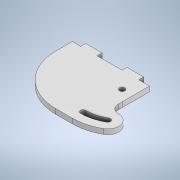
# Autodesk Inventor part: camMount
Saved by Autodesk Inventor 2020 (Build 240168000, 168)
## iProperties
Created: 2019-08-06
Part Number: camMount
Material: Generic
Document SubType Name: Modeling
Designer: n10208577
Density: 1 g/cm^3
Appearance: Default
Author: n10208577
Autodesk Inventor part; units mm, degrees
ref_plane "YZ Plane" through (0, 0, 0) normal (1, 0, 0) x (0, 1, 0)
ref_plane "XZ Plane" through (0, 0, 0) normal (0, 1, 0) x (-1, 0, 0)
ref_plane "XY Plane" through (0, 0, 0) normal (0, 0, 1) x (1, 0, 0)
sketch "Sketch1" plane through (0, 0, 0) normal (0, 1, 0) x (-1, 0, 0)
  arc A0 (9.7034, 16.3774) -> (9.7034, 19.5774) centre (9.7034, 17.9774) ccw
  circle A1 centre (9.7034, -5.5226) radius 1.6
  arc A2 (9.7034, 16.3774) -> (-1.2466, 13.4434) centre (9.7034, -5.5226) ccw
  arc A3 (9.7034, 19.5774) -> (-2.8466, 16.2146) centre (9.7034, -5.5226) ccw
  line L0 (9.7034, -15.5226) -> (3.2034, -15.5226)
  line L1 (19.7034, 24.4774) -> (9.7034, 24.4774)
  arc A4 (49.7034, -5.5226) -> (19.7034, 24.4774) centre (19.7034, -5.5226) ccw
  arc A5 (9.7034, 24.4774) -> (-5.2966, 20.4582) centre (9.7034, -5.5226) ccw
  line L2 (19.7034, -15.5226) -> (19.7034, -18.5226)
  line L3 (19.7034, -18.5226) -> (9.7034, -18.5226)
  line L4 (9.7034, -18.5226) -> (9.7034, -15.5226)
  line L5 (3.1999, 0.7949) -> (3.2034, -15.5226)
  line L6 (34.7034, -15.5226) -> (19.7034, -15.5226)
  line L7 (44.7034, -15.5226) -> (44.7034, -18.5226)
  line L8 (44.7034, -18.5226) -> (34.7034, -18.5226)
  line L9 (34.7034, -18.5226) -> (34.7034, -15.5226)
  line L10 (44.7034, -15.5226) -> (49.7034, -15.5226)
  line L11 (49.7034, -15.5226) -> (49.7034, -5.5226)
  arc A6 (-2.8466, 16.2146) -> (-1.2466, 13.4434) centre (-2.0466, 14.829) ccw
  arc A7 (-5.2966, 20.4582) -> (-2.0466, 8.329) centre (-2.0466, 14.829) ccw
  line L12 (3.1999, 0.7949) -> (3.1999, 3.329)
  line L13 (-1.8001, 8.329) -> (-2.0466, 8.329)
  arc A8 (3.1999, 3.329) -> (-1.8001, 8.329) centre (-1.8001, 3.329) ccw
  point P0 (0, 0)
  dimension "d4" = 5
  constraints: 28 end point, 17 point on circle, 9 centre point, 2 tangent, 1 coincident, 1 perpendicular, 1 vertical
  measures "d4" radius of A8
extrude "Extrusion1" add sketch "Sketch1" along normal blind 3
body "Solid1"
